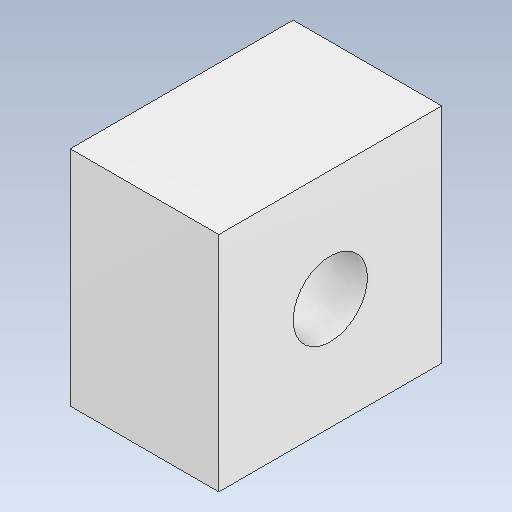
# Autodesk Inventor part: nut
Saved by Autodesk Inventor 2020 (Build 240168000, 168)
## iProperties
Created: 2021-07-04
Part Number: nut
Material: PPS Plastic
Document SubType Name: Modeling
Designer: pc
Density: 1.637 g/cm^3
Appearance: Smooth - White
Author: pc
Autodesk Inventor part; units mm, degrees
ref_plane "YZ Plane" through (0, 0, 0) normal (1, 0, 0) x (0, 1, 0)
ref_plane "XZ Plane" through (0, 0, 0) normal (0, 1, 0) x (-1, 0, 0)
ref_plane "XY Plane" through (0, 0, 0) normal (0, 0, 1) x (1, 0, 0)
sketch "Sketch1" plane through (0, 0, 0) normal (1, 0, 0) x (0, 1, 0)
  line L0 (-1.8187, -1.7212) -> (-39.9187, -1.7212)
  line L1 (-39.9187, -1.7212) -> (-39.9187, -39.8212)
  line L2 (-39.9187, -39.8212) -> (-1.8187, -39.8212)
  line L3 (-1.8187, -39.8212) -> (-1.8187, -1.7212)
  point P0 (0, 0)
  dimension "d0" = 38.1
  dimension "d1" = 38.1
  constraints: 8 end point, 2 parallel, 1 horizontal, 1 perpendicular
  measures "d0" distance of L2.end L1.end
  measures "d1" distance of L1.end L0.end
extrude "Extrusion1" add sketch "Sketch1" along normal blind 25.4
sketch "Sketch2" plane through (25.4, 0, 0) normal (1, 0, 0) x (0, 0, -1)
  circle A0 centre (20.7712, -20.8687) radius 6.35
  line L0 (39.8212, -1.8187) -> (1.7212, -1.8187) projected
  line L1 (1.7212, -1.8187) -> (1.7212, -39.9187) projected
  point P0 (0, 0)
  dimension "d4" = 12.7
  dimension "d5" = 19.05
  dimension "d6" = 19.05
  constraints: 1 centre point
  measures "d4" diameter of A0
  measures "d5" distance from line of A0.centre L0
  measures "d6" distance from line of A0.centre L1
extrude "Extrusion2" cut sketch "Sketch2" against normal blind 25.4
body "Solid1"
